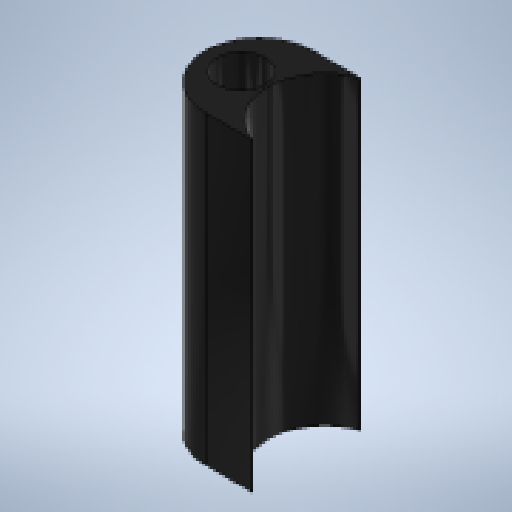
# Autodesk Inventor part: Abstandhalter
Saved by Autodesk Inventor 2024 (Build 280153000, 153)
## iProperties
Created: 2025-03-27
Part Number: Abstandhalter
Material: Generisch
Document SubType Name: Modeling
Designer: David Lill
Density: 1 g/cm^3
Appearance: Glatt - Schwarz
Author: David Lill
Autodesk Inventor part; units mm, degrees
ref_plane "YZ Plane" through (0, 0, 0) normal (1, 0, 0) x (0, 1, 0)
ref_plane "XZ Plane" through (0, 0, 0) normal (0, 1, 0) x (-1, 0, 0)
ref_plane "XY Plane" through (0, 0, 0) normal (0, 0, 1) x (1, 0, 0)
sketch "Skizze1" plane through (0, 0, 0) normal (0, 0, 1) x (1, 0, 0)
  line L0 (0, 0) -> (0, 260)
  line L1 (0, 260) -> (-3, 155)
  arc A0 (-3, 155) -> (-3, 145) centre (-3, 150) ccw
  line L2 (-3, 145) -> (0, 145)
  line L3 (0, 0) -> (0, 260)
  line L4 (0, 260) -> (-3, 210)
  arc A1 (-3, 210) -> (-3, 200) centre (-3, 205) ccw
  line L5 (-3, 200) -> (0, 200)
  line L6 (0, 130) -> (-160, 130)
  line L7 (-160, 130) -> (0, 260)
  line L8 (0, 260) -> (-160, 260)
  line L9 (-160, 260) -> (-160, 0)
  line L10 (-80, 260) -> (-80, 0)
  line L11 (-80, 0) -> (-160, 260)
  line L12 (-160, 260) -> (-160, 0)
  line L13 (-160, 0) -> (0, 0)
  line L14 (0, 0) -> (-160, 0)
  line L15 (-137.5, 31.5) -> (-158.5, 31.5)
  line L16 (-158.5, 31.5) -> (-158.5, 58.5)
  line L17 (-158.5, 58.5) -> (-137.5, 58.5)
  line L18 (-137.5, 58.5) -> (-137.5, 31.5)
  line L19 (-16.9586, 239.25) -> (-9, 239.25)
  arc A2 (-9, 239.25) -> (-9, 257.25) centre (-9, 248.25) ccw
  line L20 (-9, 257.25) -> (-16.9586, 257.25)
  arc A3 (-16.9586, 239.25) -> (-16.9586, 257.25) centre (-20, 248.25) ccw
  line L21 (-143.0414, 85.25) -> (-151, 85.25)
  arc A4 (-151, 85.25) -> (-151, 67.25) centre (-151, 76.25) ccw
  line L22 (-151, 67.25) -> (-143.0414, 67.25)
  arc A5 (-143.0414, 85.25) -> (-143.0414, 67.25) centre (-140, 76.25) ccw
  line L23 (-151, 174.75) -> (-143.0414, 174.75)
  arc A6 (-143.0414, 192.75) -> (-143.0414, 174.75) centre (-140, 183.75) ccw
  line L24 (-143.0414, 192.75) -> (-151, 192.75)
  arc A7 (-151, 192.75) -> (-151, 174.75) centre (-151, 183.75) ccw
  line L25 (-9, 20.75) -> (-16.9586, 20.75)
  arc A8 (-16.9586, 2.75) -> (-16.9586, 20.75) centre (-20, 11.75) ccw
  line L26 (-16.9586, 2.75) -> (-9, 2.75)
  arc A9 (-9, 2.75) -> (-9, 20.75) centre (-9, 11.75) ccw
  line L27 (-150, 0) -> (-150, 55)
  arc A10 (-150, 55) -> (-155, 60) centre (-155, 55) ccw
  line L28 (-155, 60) -> (-160, 60)
  line L29 (-160, 25) -> (-155, 25)
  arc A11 (-150, 20) -> (-155, 25) centre (-155, 20) ccw
  line L30 (-150, 260) -> (-150, 205)
  arc A12 (-155, 200) -> (-150, 205) centre (-155, 205) ccw
  line L31 (-155, 200) -> (-160, 200)
  line L32 (-160, 235) -> (-155, 235)
  arc A13 (-155, 235) -> (-150, 240) centre (-155, 240) ccw
  line L33 (0, 210) -> (-3, 210)
  arc A14 (-3, 210) -> (-3, 200) centre (-3, 205) ccw
  line L34 (-3, 200) -> (0, 200)
  line L35 (0, 155) -> (-3, 155)
  arc A15 (-3, 155) -> (-3, 145) centre (-3, 150) ccw
  line L36 (-3, 145) -> (0, 145)
  line L37 (-160, 145) -> (-157, 145)
  arc A16 (-157, 145) -> (-157, 155) centre (-157, 150) ccw
  line L38 (-157, 155) -> (-160, 155)
  line L39 (0, 60) -> (-3, 60)
  arc A17 (-3, 60) -> (-3, 50) centre (-3, 55) ccw
  line L40 (-3, 50) -> (0, 50)
  line L41 (0, 105) -> (-3, 105)
  arc A18 (-3, 115) -> (-3, 105) centre (-3, 110) ccw
  line L42 (-3, 115) -> (0, 115)
  line L43 (-160, 105) -> (-157, 105)
  arc A19 (-157, 105) -> (-157, 115) centre (-157, 110) ccw
  line L44 (-157, 115) -> (-160, 115)
  circle A20 centre (-20, 226.75) radius 9
  circle A21 centre (-20, 248.25) radius 9
  circle A22 centre (-20, 205.25) radius 9
  circle A23 centre (-20, 162.25) radius 9
  circle A24 centre (-20, 119.25) radius 9
  circle A25 centre (-20, 11.75) radius 9
  circle A26 centre (-20, 33.25) radius 9
  circle A27 centre (-20, 11.75) radius 9
  circle A28 centre (-20, 54.75) radius 9
  circle A29 centre (-20, 97.75) radius 9
  circle A30 centre (-20, 140.75) radius 9
  circle A31 centre (-20, 183.75) radius 9
  circle A32 centre (-40, 226.75) radius 9
  circle A33 centre (-40, 248.25) radius 9
  circle A34 centre (-40, 205.25) radius 9
  circle A35 centre (-40, 162.25) radius 9
  circle A36 centre (-40, 119.25) radius 9
  circle A37 centre (-40, 76.25) radius 9
  circle A38 centre (-40, 33.25) radius 9
  circle A39 centre (-40, 11.75) radius 9
  circle A40 centre (-40, 54.75) radius 9
  circle A41 centre (-40, 97.75) radius 9
  circle A42 centre (-40, 140.75) radius 9
  circle A43 centre (-40, 183.75) radius 9
  circle A44 centre (-60, 226.75) radius 9
  circle A45 centre (-60, 248.25) radius 9
  circle A46 centre (-60, 205.25) radius 9
  circle A47 centre (-60, 162.25) radius 9
  circle A48 centre (-60, 119.25) radius 9
  circle A49 centre (-60, 76.25) radius 9
  circle A50 centre (-60, 33.25) radius 9
  circle A51 centre (-60, 11.75) radius 9
  circle A52 centre (-60, 54.75) radius 9
  circle A53 centre (-60, 97.75) radius 9
  circle A54 centre (-60, 140.75) radius 9
  circle A55 centre (-60, 183.75) radius 9
  circle A56 centre (-80, 226.75) radius 9
  circle A57 centre (-80, 248.25) radius 9
  circle A58 centre (-80, 205.25) radius 9
  circle A59 centre (-80, 162.25) radius 9
  circle A60 centre (-80, 119.25) radius 9
  circle A61 centre (-80, 76.25) radius 9
  circle A62 centre (-80, 33.25) radius 9
  circle A63 centre (-80, 11.75) radius 9
  circle A64 centre (-80, 54.75) radius 9
  circle A65 centre (-80, 97.75) radius 9
  circle A66 centre (-80, 140.75) radius 9
  circle A67 centre (-80, 183.75) radius 9
  circle A68 centre (-100, 226.75) radius 9
  circle A69 centre (-100, 248.25) radius 9
  circle A70 centre (-100, 205.25) radius 9
  circle A71 centre (-100, 162.25) radius 9
  circle A72 centre (-100, 119.25) radius 9
  circle A73 centre (-100, 76.25) radius 9
  circle A74 centre (-100, 33.25) radius 9
  circle A75 centre (-100, 11.75) radius 9
  circle A76 centre (-100, 54.75) radius 9
  circle A77 centre (-100, 97.75) radius 9
  circle A78 centre (-100, 140.75) radius 9
  circle A79 centre (-100, 183.75) radius 9
  circle A80 centre (-120, 226.75) radius 9
  circle A81 centre (-120, 248.25) radius 9
  circle A82 centre (-120, 205.25) radius 9
  circle A83 centre (-120, 162.25) radius 9
  circle A84 centre (-120, 119.25) radius 9
  circle A85 centre (-120, 76.25) radius 9
  circle A86 centre (-120, 33.25) radius 9
  circle A87 centre (-120, 11.75) radius 9
  circle A88 centre (-120, 54.75) radius 9
  circle A89 centre (-120, 97.75) radius 9
  circle A90 centre (-120, 140.75) radius 9
  circle A91 centre (-120, 183.75) radius 9
  circle A92 centre (-140, 226.75) radius 9
  circle A93 centre (-140, 183.75) radius 9
  circle A94 centre (-140, 140.75) radius 9
  circle A95 centre (-140, 97.75) radius 9
  circle A96 centre (-140, 54.75) radius 9
  circle A97 centre (-140, 11.75) radius 9
  circle A98 centre (-140, 33.25) radius 9
  circle A99 centre (-140, 76.25) radius 9
  circle A100 centre (-140, 119.25) radius 9
  circle A101 centre (-140, 162.25) radius 9
  circle A102 centre (-140, 205.25) radius 9
  circle A103 centre (-140, 248.25) radius 9
  line L45 (0, 0) -> (0, 260)
  line L46 (-160, 0) -> (0, 0)
  line L47 (-160, 260) -> (-160, 0)
  line L48 (-160, 0) -> (0, 0)
  line L49 (0, 260) -> (-160, 260)
  line L50 (0, 130) -> (-160, 130)
  circle A104 centre (-20, 11.75) radius 9
  circle A105 centre (-3, 248.25) radius 2.5
  circle A106 centre (-154, 76.25) radius 4
  circle A107 centre (-154, 183.75) radius 4
  line L51 (-80, 260) -> (-80, 0)
  circle A108 centre (-6, 11.75) radius 4
  circle A109 centre (-6, 248.25) radius 4
  constraints: 110 centre point, 104 end point, 40 point on circle
extrude "Extrusion2" add sketch "Skizze1" along normal blind 53 contours A4 L21 A5 L22
